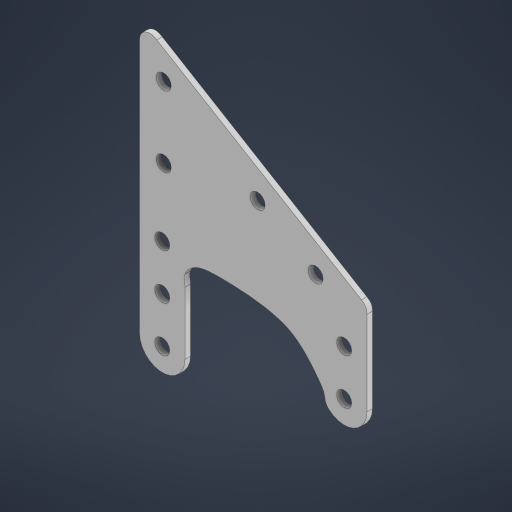
# Autodesk Inventor part: funnel
Saved by Autodesk Inventor 2023.2 (Build 272271000, 271)
## iProperties
Created: 2023-03-28
Part Number: funnel
Material: Generic
Document SubType Name: Modeling
Designer: eduar
Density: 1 g/cm^3
Appearance: Default
Author: eduar
Autodesk Inventor part; units mm, degrees
ref_plane "YZ Plane" through (0, 0, 0) normal (1, 0, 0) x (0, 1, 0)
ref_plane "XZ Plane" through (0, 0, 0) normal (0, 1, 0) x (-1, 0, 0)
ref_plane "XY Plane" through (0, 0, 0) normal (0, 0, 1) x (1, 0, 0)
sketch "Sketch1" plane through (0, 0, 0) normal (0, 0, 1) x (1, 0, 0)
  circle A0 centre (0.7751, 127) radius 2.0955
  circle A1 centre (0.7751, 139.7) radius 2.0955
  circle A2 centre (0.7751, 152.4) radius 2.0955
  circle A3 centre (51.5751, 152.4) radius 2.0955
  circle A4 centre (51.5751, 139.7) radius 2.0955
  line L0 (57.9251, 139.7) -> (57.9251, 152.4)
  line L1 (-5.5749, 127) -> (-5.5749, 197.5923)
  line L2 (57.9251, 152.4) -> (57.9251, 163.3023)
  line L3 (-0.7663, 200.3149) -> (56.3837, 166.0249)
  spline S0 degree 4 poles (56.3837, 166.0249) (56.7408, 165.8106) (57.455, 165.3821) (57.9251, 164.5517) (57.9251, 163.7188) (57.9251, 163.3023) knots 0 0 0 0 0 0.5 1 1 1 1 1
  spline S1 degree 4 poles (-0.7663, 200.3149) (-1.5089, 200.7604) (-2.9939, 201.6514) (-5.5749, 200.1901) (-5.5749, 198.4583) (-5.5749, 197.5923) knots 0 0 0 0 0 0.5 1 1 1 1 1
  line L4 (7.1251, 147.6375) -> (8.9582, 151.7525) construction
  line L5 (8.9582, 151.7525) -> (16.6389, 151.7525) construction
  line L6 (16.6389, 151.7525) -> (25.4, 151.7525) construction
  line L7 (25.4, 151.7525) -> (33.3375, 150.3172) construction
  line L8 (33.3375, 150.3172) -> (39.6875, 147.6375) construction
  line L9 (39.6875, 147.6375) -> (45.2251, 139.7) construction
  spline S2 degree 4 poles (7.1251, 147.6375) (8.9582, 151.7525) (16.6389, 151.7525) (25.4, 151.7525) (33.3375, 150.3172) (39.6875, 147.6375) (45.2251, 139.7) knots 1 1 1 1 1 2 3 4 4 4 4 4
  arc A5 (-5.5749, 127) -> (7.1251, 127) centre (0.7751, 127) ccw
  line L10 (7.1251, 127) -> (7.1251, 144.4625)
  spline S3 degree 4 poles (7.1251, 144.4625) (7.1251, 144.8594) (7.1251, 145.6531) (6.6738, 146.4787) (6.9567, 147.2593) (7.1251, 147.6375) knots 0 0 0 0 0 0.5 1 1 1 1 1
  arc A6 (47.3211, 134.9856) -> (57.9251, 139.7) centre (51.5751, 139.7) ccw
  spline S4 degree 4 poles (47.3211, 134.9856) (46.8217, 135.4363) (45.9501, 136.4787) (46.3422, 138.0988) (45.5975, 139.1663) (45.2251, 139.7) knots 0 0 0 0 0 0.5 1 1 1 1 1
  circle A7 centre (1.1822, 191.2221) radius 2.0955
  circle A8 centre (27.4016, 175.4904) radius 2.0955
  circle A9 centre (43.5997, 165.7716) radius 2.0955
  circle A10 centre (1.1822, 171.45) radius 2.0955
  point P0 (0, 0)
  point P1 (-5.5749, 203.2)
  point P2 (57.9251, 165.1)
  dimension "d7" = 50.8
  dimension "d8" = 12.7
  dimension "d10" = 6.35
  dimension "d13" = 4.191
  dimension "d14" = 4.191
  dimension "d15" = 4.191
  dimension "d16" = 4.191
  dimension "d17" = 4.191
  dimension "d18" = 4.191
  dimension "d19" = 4.191
  dimension "d20" = 4.191
  dimension "d21" = 4.191
  constraints: 11 centre point, 10 end point, 5 point on line, 5 vertical, 4 point on circle, 2 coincident, 1 horizontal, 33 other
  measures "d7" vertical distance of A2.centre point (-5.575, 203.2)
  measures "d8" vertical distance of A3.centre point (57.925, 165.1)
  measures "d10" radius of A5
  measures "d13" diameter of A7
  measures "d14" diameter of A8
  measures "d15" diameter of A9
  measures "d16" diameter of A2
  measures "d17" diameter of A1
  measures "d18" diameter of A0
  measures "d19" diameter of A3
  measures "d20" diameter of A4
  measures "d21" diameter of A10
extrude "Extrusion1" add sketch "Sketch1" along normal blind 1.524
body "Solid1"
